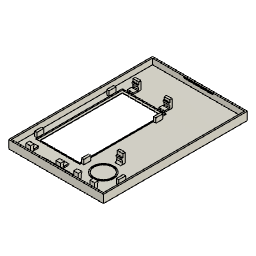
epaper Outer Case Top (Autodesk Fusion 360 design; units mm, degrees)
Autodesk Fusion 360 part; units mm, degrees
sketch "Sketch2" plane through (0, 0, 0) normal (0, 0, 1) x (1, 0, 0)
  line L0 (0, 0) -> (82, 0)
  line L1 (82, 0) -> (82, 124.4)
  line L2 (82, 124.4) -> (0, 124.4)
  line L3 (0, 124.4) -> (0, 0)
  dimension "d135" = 124.4
  dimension "d136" = 82
  constraint horizontal L0
  constraint vertical L1
  constraint horizontal L2
  constraint vertical L3
  constraint coincident L0.start L3.end
  measures "d135" distance of L0.start L2.end
  measures "d136" distance of L0.start L0.end
extrude "Extrude4" add sketch "Sketch2" along normal blind 2
sketch "Sketch3" plane through (0, 0, 2) normal (0, 0, 1) x (-1, 0, 0)
  line L0 (0, -124.4) -> (0, 0)
  line L1 (0, 0) -> (-82, 0)
  line L2 (-82, 0) -> (-82, -124.4)
  line L3 (-82, -124.4) -> (0, -124.4)
  line L4 (-1.25, -1.25) -> (-80.75, -1.25)
  line L5 (-80.75, -1.25) -> (-80.75, -123.15)
  line L6 (-80.75, -123.15) -> (-1.25, -123.15)
  line L7 (-1.25, -123.15) -> (-1.25, -1.25)
  line L8 (-51.575, -4.675) -> (-55.575, -4.675)
  line L9 (-55.575, -4.675) -> (-55.575, -7.175)
  line L10 (-55.575, -7.175) -> (-51.575, -7.175)
  line L11 (-51.575, -7.175) -> (-51.575, -4.675)
  line L12 (-65.625, -4.675) -> (-69.625, -4.675)
  line L13 (-69.625, -4.675) -> (-69.625, -7.175)
  line L14 (-69.625, -7.175) -> (-65.625, -7.175)
  line L15 (-65.625, -7.175) -> (-65.625, -4.675)
  line L16 (-58.1, -35.275) -> (-63.1, -35.275)
  line L17 (-63.1, -35.275) -> (-63.1, -37.775)
  line L18 (-63.1, -37.775) -> (-58.1, -37.775)
  line L19 (-58.1, -37.775) -> (-58.1, -35.275)
  line L20 (-74.75, -24.5) -> (-76.75, -24.5)
  line L21 (-76.75, -24.5) -> (-76.75, -18.5)
  line L22 (-76.75, -18.5) -> (-74.75, -18.5)
  line L23 (-74.75, -18.5) -> (-74.75, -24.5)
  line L24 (-44.45, -24.5) -> (-46.45, -24.5)
  line L25 (-46.45, -24.5) -> (-46.45, -18.5)
  line L26 (-46.45, -18.5) -> (-44.45, -18.5)
  line L27 (-44.45, -18.5) -> (-44.45, -24.5)
  circle A0 centre (-60.6, -21.25) radius 8.0623
  circle A1 centre (-60.6, -21.25) radius 9.0623
  line L28 (0, 0) -> (-82, 0)
  line L29 (0, -124.4) -> (0, 0)
  line L30 (-80.75, -110) -> (-80.75, -72)
  line L31 (-46.45, -80.825) -> (-44.45, -80.825)
  line L32 (-44.45, -80.825) -> (-44.45, -86.825)
  line L33 (-44.45, -86.825) -> (-46.45, -86.825)
  line L34 (-46.45, -86.825) -> (-46.45, -80.825)
  line L35 (-3.95, -86.825) -> (-5.95, -86.825)
  line L36 (-5.95, -86.825) -> (-5.95, -80.825)
  line L37 (-5.95, -80.825) -> (-3.95, -80.825)
  line L38 (-3.95, -80.825) -> (-3.95, -86.825)
  line L39 (-3.95, -24.5) -> (-5.95, -24.5)
  line L40 (-5.95, -24.5) -> (-5.95, -18.5)
  line L41 (-5.95, -18.5) -> (-3.95, -18.5)
  line L42 (-3.95, -18.5) -> (-3.95, -24.5)
  line L43 (-10.2, -7.175) -> (-14.2, -7.175)
  line L44 (-14.2, -7.175) -> (-14.2, -4.675)
  line L45 (-14.2, -4.675) -> (-10.2, -4.675)
  line L46 (-10.2, -4.675) -> (-10.2, -7.175)
  line L47 (-36.2, -7.175) -> (-40.2, -7.175)
  line L48 (-40.2, -7.175) -> (-40.2, -4.675)
  line L49 (-40.2, -4.675) -> (-36.2, -4.675)
  line L50 (-36.2, -4.675) -> (-36.2, -7.175)
  line L51 (-10.2, -99.325) -> (-15.2, -99.325)
  line L52 (-15.2, -99.325) -> (-15.2, -97.075)
  line L53 (-15.2, -97.075) -> (-10.2, -97.075)
  line L54 (-10.2, -97.075) -> (-10.2, -99.325)
  line L55 (-37.2, -99.325) -> (-42.2, -99.325)
  line L56 (-42.2, -99.325) -> (-42.2, -97.075)
  line L57 (-42.2, -97.075) -> (-37.2, -97.075)
  line L58 (-37.2, -97.075) -> (-37.2, -99.325)
  line L59 (-10.2, -8.175) -> (-14.2, -8.175)
  line L60 (-14.2, -8.175) -> (-14.2, -11.675)
  line L61 (-14.2, -11.675) -> (-10.2, -11.675)
  line L62 (-10.2, -11.675) -> (-10.2, -8.175)
  line L63 (-40.2, -8.175) -> (-36.2, -8.175)
  line L64 (-36.2, -8.175) -> (-36.2, -11.675)
  line L65 (-36.2, -11.675) -> (-40.2, -11.675)
  line L66 (-40.2, -11.675) -> (-40.2, -8.175)
  line L67 (-10.2, -96.075) -> (-15.2, -96.075)
  line L68 (-15.2, -96.075) -> (-15.2, -92.575)
  line L69 (-15.2, -92.575) -> (-10.2, -92.575)
  line L70 (-10.2, -92.575) -> (-10.2, -96.075)
  line L71 (-42.2, -96.075) -> (-37.2, -96.075)
  line L72 (-37.2, -96.075) -> (-37.2, -92.575)
  line L73 (-37.2, -92.575) -> (-42.2, -92.575)
  line L74 (-42.2, -92.575) -> (-42.2, -96.075)
  line L75 (-8.2, -90.175) -> (-42.2, -90.175)
  line L76 (-42.2, -90.175) -> (-42.2, -19.175)
  line L77 (-42.2, -19.175) -> (-8.2, -19.175)
  line L78 (-8.2, -19.175) -> (-8.2, -90.175)
  line L79 (-6.2, -17.175) -> (-6.2, -92.175)
  line L80 (-6.2, -92.175) -> (-44.2, -92.175)
  line L81 (-44.2, -92.175) -> (-44.2, -17.175)
  line L82 (-44.2, -17.175) -> (-6.2, -17.175)
  dimension "d82" = -1.25
  dimension "d87" = 4
  dimension "d88" = 2.5
  dimension "d89" = 4
  dimension "d90" = 2.5
  dimension "d93" = 5
  dimension "d94" = 2.5
  dimension "d96" = 2
  dimension "d97" = 6
  dimension "d98" = 2
  dimension "d99" = 6
  dimension "d102" = 11.65
  dimension "d103" = 28.3
  dimension "d104" = 1
  dimension "d122" = 14.15
  dimension "d129" = 79.5
  dimension "d131" = 20
  dimension "d137" = 82
  dimension "d169" = 28.1
  dimension "d170" = 14.025
  dimension "d193" = 124.4
  dimension "d213" = 20.15
  dimension "d216" = 5.025
  dimension "d217" = 10.05
  dimension "d222" = 2
  dimension "d223" = 6
  dimension "d224" = 2
  dimension "d225" = 6
  dimension "d226" = 2
  dimension "d227" = 6
  dimension "d228" = 38.5
  dimension "d229" = 22
  dimension "d230" = 8.25
  dimension "d231" = 2.5
  dimension "d232" = 2.5
  dimension "d234" = 5
  dimension "d235" = 2.25
  dimension "d236" = 89.9
  dimension "d237" = 4
  dimension "d238" = 4
  dimension "d239" = 2.25
  dimension "d240" = 5
  dimension "d241" = 22
  dimension "d242" = 10.25
  dimension "d243" = 4
  dimension "d244" = 3.5
  dimension "d245" = 4
  dimension "d246" = 3.5
  dimension "d247" = 5
  dimension "d248" = 3.5
  dimension "d249" = 5
  dimension "d250" = 3.5
  dimension "d251" = 1
  dimension "d252" = 1
  dimension "d257" = 34
  dimension "d258" = 71
  dimension "d259" = 12
  dimension "d260" = 2.25
  dimension "d263" = -2
  constraint horizontal L8
  constraint vertical L9
  constraint horizontal L10
  constraint vertical L11
  constraint horizontal L12
  constraint vertical L13
  constraint horizontal L14
  constraint vertical L15
  constraint horizontal L16
  constraint vertical L17
  constraint horizontal L18
  constraint vertical L19
  constraint horizontal L10.end L14.end
  constraint horizontal L20
  constraint vertical L21
  constraint horizontal L22
  constraint vertical L23
  constraint horizontal L24
  constraint vertical L25
  constraint horizontal L26
  constraint vertical L27
  constraint horizontal L20.start L24.end
  constraint vertical L30
  constraint coincident L5 L30.end
  constraint horizontal L31
  constraint vertical L32
  constraint horizontal L33
  constraint vertical L34
  constraint collinear L27 L32
  constraint horizontal L35
  constraint vertical L36
  constraint horizontal L37
  constraint vertical L38
  constraint horizontal L39
  constraint vertical L40
  constraint horizontal L41
  constraint vertical L42
  constraint collinear L38 L42
  constraint collinear L24 L39
  constraint collinear L33 L35
  constraint horizontal L43
  constraint vertical L44
  constraint horizontal L45
  constraint vertical L46
  constraint horizontal L47
  constraint vertical L48
  constraint horizontal L49
  constraint vertical L50
  constraint collinear L43 L47
  constraint horizontal L51
  constraint vertical L52
  constraint horizontal L53
  constraint vertical L54
  constraint collinear L46 L54
  constraint horizontal L55
  constraint vertical L56
  constraint horizontal L57
  constraint vertical L58
  constraint collinear L51 L55
  constraint horizontal L59
  constraint vertical L60
  constraint horizontal L61
  constraint vertical L62
  constraint horizontal L63
  constraint vertical L64
  constraint horizontal L65
  constraint vertical L66
  constraint horizontal L67
  constraint vertical L68
  constraint horizontal L69
  constraint vertical L70
  constraint horizontal L71
  constraint vertical L72
  constraint horizontal L73
  constraint vertical L74
  constraint collinear L67 L71
  constraint collinear L59 L63
  constraint collinear L46 L62
  constraint collinear L48 L66
  constraint collinear L54 L70
  constraint collinear L56 L74
  constraint horizontal L75
  constraint vertical L76
  constraint horizontal L77
  constraint vertical L78
  constraint collinear L8 L45
  measures "d87" distance of L8.start L8.end
  measures "d88" distance of L8.start L10.end
  measures "d89" distance of L12.start L12.end
  measures "d90" distance of L12.start L14.end
  measures "d93" distance of L16.start L16.end
  measures "d94" distance of L16.start L18.end
  measures "d96" distance of L20.start L20.end
  measures "d97" distance of L20.start L22.end
  measures "d98" distance of L24.start L24.end
  measures "d99" distance of L24.start L26.end
  measures "d102" distance of L17 L23
  measures "d103" distance of L23 L25
  measures "d122" distance of L25 A0.centre
  measures "d129" distance of L5 L7
  measures "d131" distance of L4 A0.centre
  measures "d137" distance of L0.end L1.end
  measures "d169" distance of L14 L16
  measures "d170" distance of L16 A0.centre
  measures "d193" distance of L0.start L0.end
  measures "d213" distance of L5 A0.centre
  measures "d216" distance of L9 A0.centre
  measures "d217" distance of L9 L15
  measures "d222" distance of L31.start L31.end
  measures "d223" distance of L31.start L33.end
  measures "d224" distance of L35.start L35.end
  measures "d225" distance of L35.start L37.end
  measures "d226" distance of L39.start L39.end
  measures "d227" distance of L39.start L41.end
  measures "d228" distance of L32 L36
  measures "d229" distance of L44 L50
  measures "d230" distance of L27 L50
  measures "d231" distance of L43.start L45.end
  measures "d232" distance of L47.end L48.end
  measures "d234" distance of L51.start L51.end
  measures "d235" distance of L51.start L53.end
  measures "d236" distance of L43 L53
  measures "d237" distance of L44.end L45.end
  measures "d238" distance of L48.end L49.end
  measures "d239" distance of L55.start L57.end
  measures "d240" distance of L55.start L55.end
  measures "d241" distance of L52 L58
  measures "d242" distance of L33 L56.end
  measures "d243" distance of L59.start L59.end
  measures "d244" distance of L59.start L61.end
  measures "d245" distance of L63.start L63.end
  measures "d246" distance of L63.start L65.end
  measures "d247" distance of L67.start L67.end
  measures "d248" distance of L67.start L69.end
  measures "d249" distance of L71.start L71.end
  measures "d250" distance of L71.start L73.end
  measures "d251" distance of L53 L67
  measures "d252" distance of L43 L59
  measures "d257" distance of L76 L78
  measures "d258" distance of L75 L77
  measures "d259" distance of L43 L77
  measures "d260" distance of L36 L78
extrude "Extrude26" cut sketch "Sketch3" against normal blind 1 contours L79 L80 L81 L82
extrude "Extrude25" cut sketch "Sketch3" against normal blind 4 contours L75 L76 L77 L78
extrude "Extrude24" add sketch "Sketch3" along normal blind 3 contours L43 L44 L45 L46 | L47 L48 L49 L50 | L51 L52 L53 L54 | L55 L56 L57 L58
extrude "Extrude23" add sketch "Sketch3" along normal blind 1.2 contours L59 L60 L61 L62 | L63 L64 L65 L66 | L67 L68 L69 L70 | L71 L72 L73 L74
extrude "Extrude11" add sketch "Sketch3" along normal blind 0.3 contours A1
extrude "Extrude12" add sketch "Sketch3" along normal blind 4 contours L20 L21 L22 L23 | L24 L25 L26 L27 | L31 L32 L33 L34 | L35 L36 L37 L38 | L39 L40 L41 L42
extrude "Extrude13" add sketch "Sketch3" along normal blind 3.23 contours L8 L9 L10 L11 | L12 L13 L14 L15 | L16 L17 L18 L19
sketch "Sketch7" plane through (0, 0, 5.23) normal (0, 0, 1) x (-1, 0, 0)
  line L0 (-58.1, -37.775) -> (-63.1, -37.775)
  line L1 (-63.1, -37.775) -> (-63.1, -34.775)
  line L2 (-63.1, -34.775) -> (-58.1, -34.775)
  line L3 (-58.1, -34.775) -> (-58.1, -37.775)
  line L4 (-51.575, -4.675) -> (-55.575, -4.675)
  line L5 (-55.575, -4.675) -> (-55.575, -7.675)
  line L6 (-55.575, -7.675) -> (-51.575, -7.675)
  line L7 (-51.575, -7.675) -> (-51.575, -4.675)
  line L8 (-65.625, -4.675) -> (-69.625, -4.675)
  line L9 (-69.625, -4.675) -> (-69.625, -7.675)
  line L10 (-69.625, -7.675) -> (-65.625, -7.675)
  line L11 (-65.625, -7.675) -> (-65.625, -4.675)
  line L12 (-58.1, -37.775) -> (-58.1, -35.275)
  line L13 (-58.1, -35.275) -> (-63.1, -35.275)
  line L14 (-63.1, -35.275) -> (-63.1, -37.775)
  line L15 (-63.1, -37.775) -> (-58.1, -37.775)
  line L16 (-65.625, -7.175) -> (-65.625, -4.675)
  line L17 (-65.625, -4.675) -> (-69.625, -4.675)
  line L18 (-69.625, -4.675) -> (-69.625, -7.175)
  line L19 (-69.625, -7.175) -> (-65.625, -7.175)
  line L20 (-51.575, -7.175) -> (-51.575, -4.675)
  line L21 (-51.575, -4.675) -> (-55.575, -4.675)
  line L22 (-55.575, -4.675) -> (-55.575, -7.175)
  line L23 (-55.575, -7.175) -> (-51.575, -7.175)
  point P0 (-58.1, -37.775)
  point P1 (-51.575, -4.675)
  point P2 (-65.625, -4.675)
  point P3 (-63.1, -37.775)
  dimension "d112" = 3
  dimension "d113" = 4
  dimension "d114" = 3
  dimension "d115" = 4
  dimension "d116" = 3
  constraint horizontal L0
  constraint vertical L1
  constraint horizontal L2
  constraint vertical L3
  constraint horizontal L4
  constraint vertical L5
  constraint horizontal L6
  constraint vertical L7
  constraint horizontal L8
  constraint vertical L9
  constraint horizontal L10
  constraint vertical L11
  constraint coincident P0 L0.start
  constraint coincident P1 L4.start
  constraint coincident P2 L8.start
  constraint coincident P3 L0.end
  measures "d112" distance of P0 L2.end
  measures "d113" distance of P1 L4.end
  measures "d114" distance of P1 L6.end
  measures "d115" distance of P2 L8.end
  measures "d116" distance of P2 L10.end
extrude "Extrude14" add sketch "Sketch7" along normal blind 1.8
extrude "Extrude10" add sketch "Sketch3" along normal blind 5 contours L0 L1 L2 L3 L28 L29
sketch "Sketch12" plane through (0, 0, 7.03) normal (0, 0, 1) x (-1, 0, 0)
  line L0 (-58.1, -34.775) -> (-63.1, -34.775)
  line L1 (-63.1, -34.775) -> (-63.1, -37.775)
  line L2 (-63.1, -37.775) -> (-58.1, -37.775)
  line L3 (-58.1, -37.775) -> (-58.1, -34.775)
  line L4 (-58.1, -37.775) -> (-63.1, -37.775)
  line L5 (-63.1, -37.775) -> (-63.1, -35.775)
  line L6 (-63.1, -35.775) -> (-58.1, -35.775)
  line L7 (-58.1, -35.775) -> (-58.1, -37.775)
  dimension "d160" = 2
  constraint horizontal L4
  constraint vertical L5
  constraint horizontal L6
  constraint vertical L7
  constraint coincident L2.end L3.start
  constraint coincident L1.end L2.start
  measures "d160" distance of L2.end L6.end
extrude "Extrude18" add sketch "Sketch12" along normal blind 3 contours L1 L2 L3 L4 L5 L6 L7
chamfer "Chamfer5" distance 0.5 angle 45 3 edges at (60.6, 34.775, 5.23) (53.575, 7.675, 5.23) (67.625, 7.675, 5.23)
sketch "Sketch19" plane through (0, 0, 5) normal (0, 0, 1) x (-1, 0, 0)
  line L0 (-10.2, -4.675) -> (-14.2, -4.675)
  line L1 (-14.2, -4.675) -> (-14.2, -7.175)
  line L2 (-14.2, -7.175) -> (-10.2, -7.175)
  line L3 (-10.2, -7.175) -> (-10.2, -4.675)
  line L4 (-10.2, -4.675) -> (-14.2, -4.675)
  line L5 (-14.2, -4.675) -> (-14.2, -7.775)
  line L6 (-14.2, -7.775) -> (-10.2, -7.775)
  line L7 (-10.2, -7.775) -> (-10.2, -4.675)
  dimension "d267" = 4
  dimension "d268" = 3.1
  constraint horizontal L4
  constraint vertical L5
  constraint horizontal L6
  constraint vertical L7
  constraint coincident L0.start L3.end
  measures "d267" distance of L0.start L0.end
  measures "d268" distance of L0.start L6.end
extrude "Extrude27" add sketch "Sketch19" along normal blind 2
sketch "Sketch20" plane through (0, 0, 5) normal (0, 0, 1) x (-1, 0, 0)
  line L0 (-36.2, -4.675) -> (-40.2, -4.675)
  line L1 (-40.2, -4.675) -> (-40.2, -7.175)
  line L2 (-40.2, -7.175) -> (-36.2, -7.175)
  line L3 (-36.2, -7.175) -> (-36.2, -4.675)
  line L4 (-36.2, -4.675) -> (-40.2, -4.675)
  line L5 (-40.2, -4.675) -> (-40.2, -7.775)
  line L6 (-40.2, -7.775) -> (-36.2, -7.775)
  line L7 (-36.2, -7.775) -> (-36.2, -4.675)
  dimension "d271" = 4
  dimension "d272" = 3.1
  constraint horizontal L4
  constraint vertical L5
  constraint horizontal L6
  constraint vertical L7
  constraint coincident L0.start L3.end
  measures "d271" distance of L0.start L0.end
  measures "d272" distance of L0.start L6.end
extrude "Extrude28" add sketch "Sketch20" along normal blind 2
sketch "Sketch21" plane through (0, 0, 5) normal (0, 0, 1) x (-1, 0, 0)
  line L0 (-10.2, -97.075) -> (-15.2, -97.075)
  line L1 (-15.2, -97.075) -> (-15.2, -99.325)
  line L2 (-15.2, -99.325) -> (-10.2, -99.325)
  line L3 (-10.2, -99.325) -> (-10.2, -97.075)
  line L4 (-10.2, -99.325) -> (-15.2, -99.325)
  line L5 (-15.2, -99.325) -> (-15.2, -96.475)
  line L6 (-15.2, -96.475) -> (-10.2, -96.475)
  line L7 (-10.2, -96.475) -> (-10.2, -99.325)
  dimension "d275" = 5
  dimension "d276" = 2.85
  constraint horizontal L4
  constraint vertical L5
  constraint horizontal L6
  constraint vertical L7
  constraint coincident L2.end L3.start
  measures "d275" distance of L2.end L1.end
  measures "d276" distance of L2.end L6.end
extrude "Extrude29" add sketch "Sketch21" along normal blind 2
sketch "Sketch22" plane through (0, 0, 5) normal (0, 0, 1) x (-1, 0, 0)
  line L0 (-37.2, -97.075) -> (-42.2, -97.075)
  line L1 (-42.2, -97.075) -> (-42.2, -99.325)
  line L2 (-42.2, -99.325) -> (-37.2, -99.325)
  line L3 (-37.2, -99.325) -> (-37.2, -97.075)
  line L4 (-37.2, -99.325) -> (-42.2, -99.325)
  line L5 (-42.2, -99.325) -> (-42.2, -96.475)
  line L6 (-42.2, -96.475) -> (-37.2, -96.475)
  line L7 (-37.2, -96.475) -> (-37.2, -99.325)
  dimension "d279" = 5
  dimension "d280" = 2.85
  constraint horizontal L4
  constraint vertical L5
  constraint horizontal L6
  constraint vertical L7
  constraint coincident L2.end L3.start
  measures "d279" distance of L2.end L1.end
  measures "d280" distance of L2.end L6.end
extrude "Extrude30" add sketch "Sketch22" along normal blind 2
chamfer "Chamfer9" distance 0.6 angle 45 2 edges at (12.2, 7.775, 5) (38.2, 7.775, 5)
chamfer "Chamfer10" distance 0.6 angle 45 2 edges at (12.7, 96.475, 5) (39.7, 96.475, 5)
sketch "Sketch23" plane through (0, 0, 7) normal (0, 0, 1) x (-1, 0, 0)
  line L0 (-10.2, -96.475) -> (-15.2, -96.475)
  line L1 (-15.2, -96.475) -> (-15.2, -99.325)
  line L2 (-15.2, -99.325) -> (-10.2, -99.325)
  line L3 (-10.2, -99.325) -> (-10.2, -96.475)
  line L4 (-10.2, -99.325) -> (-15.2, -99.325)
  line L5 (-15.2, -99.325) -> (-15.2, -97.325)
  line L6 (-15.2, -97.325) -> (-10.2, -97.325)
  line L7 (-10.2, -97.325) -> (-10.2, -99.325)
  dimension "d284" = 5
  dimension "d285" = 2
  constraint horizontal L4
  constraint vertical L5
  constraint horizontal L6
  constraint vertical L7
  constraint coincident L2.end L3.start
  measures "d284" distance of L2.end L1.end
  measures "d285" distance of L2.end L6.end
extrude "Extrude31" add sketch "Sketch23" along normal blind 2 contours L1 L2 L3 L4 L5 L6 L7
sketch "Sketch24" plane through (0, 0, 7) normal (0, 0, 1) x (-1, 0, 0)
  line L0 (-37.2, -96.475) -> (-42.2, -96.475)
  line L1 (-42.2, -96.475) -> (-42.2, -99.325)
  line L2 (-42.2, -99.325) -> (-37.2, -99.325)
  line L3 (-37.2, -99.325) -> (-37.2, -96.475)
  line L4 (-37.2, -99.325) -> (-42.2, -99.325)
  line L5 (-42.2, -99.325) -> (-42.2, -97.325)
  line L6 (-42.2, -97.325) -> (-37.2, -97.325)
  line L7 (-37.2, -97.325) -> (-37.2, -99.325)
  dimension "d288" = 5
  dimension "d289" = 2
  constraint horizontal L4
  constraint vertical L5
  constraint horizontal L6
  constraint vertical L7
  constraint coincident L2.end L3.start
  measures "d288" distance of L2.end L1.end
  measures "d289" distance of L2.end L6.end
extrude "Extrude32" add sketch "Sketch24" along normal blind 2 contours L1 L2 L3 L4 L5 L6 L7
sketch "Sketch8" plane through (0, 0, 0) normal (0, 0, -1) x (1, 0, 0)
  line L0 (0, 0) -> (0, -124.4)
  line L1 (0, -124.4) -> (82, -124.4)
  line L2 (82, -124.4) -> (82, 0)
  line L3 (82, 0) -> (0, 0)
  line L4 (57.8279, -10.7958) -> (57.8279, -104.0301) construction
  line L5 (57.8279, -104.0301) -> (69.8279, -104.0301) construction
  line L6 (69.8279, -104.0301) -> (69.8279, -10.7958) construction
  line L7 (69.8279, -10.7958) -> (57.8279, -10.7958) construction
  line L8 (42.2, -19.175) -> (42.2, -90.175)
  line L9 (42.2, -90.175) -> (8.2, -90.175)
  line L10 (8.2, -90.175) -> (8.2, -19.175)
  line L11 (8.2, -19.175) -> (42.2, -19.175)
  text T0 "Ferg Data Logger" font "Arial" height 12 align ink ink in box 0 x 0 at (57.8279, -10.7958) x (0, -1) y (1, 0) spacing 1 height is em
  constraint perpendicular L4 L5
  constraint parallel L4 L6
  constraint parallel L5 L7
extrude "Extrude16" cut sketch "Sketch8" against normal blind 0.5 text T0
sketch "Sketch10" plane through (0, 123.15, 0) normal (0, -1, 0) x (1, 0, 0)
  line L0 (1.25, 2) -> (80.75, 2)
  line L1 (80.75, 2) -> (80.75, 7)
  line L2 (80.75, 7) -> (1.25, 7)
  line L3 (1.25, 7) -> (1.25, 2)
  line L4 (28.5, 7) -> (53.5, 7)
  line L5 (53.5, 7) -> (53.5, 5.6)
  line L6 (53.5, 5.6) -> (28.5, 5.6)
  line L7 (28.5, 5.6) -> (28.5, 7)
  dimension "d139" = 25
  dimension "d140" = 1.4
  dimension "d141" = 79.5
  dimension "d142" = 27.25
  constraint horizontal L4
  constraint vertical L5
  constraint horizontal L6
  constraint vertical L7
  constraint coincident L2 L4.start
  measures "d139" distance of L4.start L4.end
  measures "d140" distance of L4.start L6.end
  measures "d141" distance of L1.end L2.end
  measures "d142" distance of L3 L7
revolve "Revolve1" add sketch "Sketch10" angle 25 about axis through (53.5, 123.15, 5.6) along (1, 0, 0) contours L2 L4 L5 L6 L7
sketch "Sketch11" plane through (0, 1.25, 0) normal (0, 1, 0) x (-1, 0, 0)
  line L0 (-80.75, 2) -> (-1.25, 2)
  line L1 (-1.25, 2) -> (-1.25, 7)
  line L2 (-1.25, 7) -> (-80.75, 7)
  line L3 (-53.5, 7) -> (-28.5, 7)
  line L4 (-28.5, 7) -> (-28.5, 5.6)
  line L5 (-28.5, 5.6) -> (-53.5, 5.6)
  line L6 (-53.5, 5.6) -> (-53.5, 7)
  line L7 (-80.75, 7) -> (-80.75, 2)
  dimension "d144" = 25
  dimension "d145" = 1.4
  dimension "d146" = 79.5
  dimension "d147" = 27.25
  constraint horizontal L3
  constraint vertical L4
  constraint horizontal L5
  constraint vertical L6
  constraint coincident L2 L3.start
  measures "d144" distance of L3.start L3.end
  measures "d145" distance of L3.start L5.end
  measures "d146" distance of L1.end L2.end
  measures "d147" distance of L1 L4
revolve "Revolve2" add sketch "Sketch11" angle 25 about axis through (28.5, 1.25, 5.6) along (-1, 0, 0) contours L2 L3 L4 L5 L6
fillet "Fillet3" radius 1.5 1 edges at (60.6, 35.275, 2)
fillet "Fillet3" radius 1.5 2 edges at (12.7, 97.075, 2) (39.7, 97.075, 2)
fillet "Fillet3" radius 1.5 2 edges at (12.2, 7.175, 2) (38.2, 7.175, 2)
sketch "Sketch18" plane through (0, 0, 2) normal (0, 0, 1) x (-1, 0, 0)
  line L0 (-58.1, -33.775) -> (-58.1, -37.775)
  line L1 (-58.1, -37.775) -> (-63.1, -37.775)
  line L2 (-63.1, -37.775) -> (-63.1, -33.775)
  line L3 (-63.1, -33.775) -> (-58.1, -33.775)
  line L4 (-1.25, -1.25) -> (-80.75, -1.25)
  line L5 (-80.75, -1.25) -> (-80.75, -123.15)
  line L6 (-80.75, -123.15) -> (-1.25, -123.15)
  line L7 (-1.25, -123.15) -> (-1.25, -1.25)
  line L8 (-65.625, -7.175) -> (-69.625, -7.175)
  line L9 (-69.625, -7.175) -> (-69.625, -4.675)
  line L10 (-69.625, -4.675) -> (-65.625, -4.675)
  line L11 (-65.625, -4.675) -> (-65.625, -7.175)
  line L12 (-51.575, -7.175) -> (-55.575, -7.175)
  line L13 (-55.575, -7.175) -> (-55.575, -4.675)
  line L14 (-55.575, -4.675) -> (-51.575, -4.675)
  line L15 (-51.575, -4.675) -> (-51.575, -7.175)
  line L16 (-74.75, -18.5) -> (-74.75, -24.5)
  line L17 (-74.75, -24.5) -> (-76.75, -24.5)
  line L18 (-76.75, -24.5) -> (-76.75, -18.5)
  line L19 (-76.75, -18.5) -> (-74.75, -18.5)
  line L20 (-44.45, -18.5) -> (-44.45, -24.5)
  line L21 (-44.45, -24.5) -> (-46.45, -24.5)
  line L22 (-46.45, -24.5) -> (-46.45, -18.5)
  line L23 (-46.45, -18.5) -> (-44.45, -18.5)
  circle A0 centre (-60.6, -21.25) radius 9.0623
  line L24 (-5.2392, -108.6182) -> (-65.3716, -108.6182)
  line L25 (-65.3716, -108.6182) -> (-65.3716, -3.4636)
  line L26 (-65.3716, -3.4636) -> (-5.2392, -3.4636)
  line L27 (-5.2392, -3.4636) -> (-5.2392, -108.6182)
  line L28 (-46.45, -86.825) -> (-46.45, -80.825)
  line L29 (-46.45, -80.825) -> (-44.45, -80.825)
  line L30 (-44.45, -80.825) -> (-44.45, -86.825)
  line L31 (-44.45, -86.825) -> (-46.45, -86.825)
  line L32 (-3.95, -80.825) -> (-3.95, -86.825)
  line L33 (-3.95, -86.825) -> (-5.95, -86.825)
  line L34 (-5.95, -86.825) -> (-5.95, -80.825)
  line L35 (-5.95, -80.825) -> (-3.95, -80.825)
  line L36 (-3.95, -18.5) -> (-3.95, -24.5)
  line L37 (-3.95, -24.5) -> (-5.95, -24.5)
  line L38 (-5.95, -24.5) -> (-5.95, -18.5)
  line L39 (-5.95, -18.5) -> (-3.95, -18.5)
  line L40 (-42.2, -92.575) -> (-37.2, -92.575)
  line L41 (-37.2, -92.575) -> (-37.2, -96.075)
  line L42 (-42.2, -96.075) -> (-42.2, -92.575)
  line L43 (-10.2, -11.675) -> (-14.2, -11.675)
  line L44 (-14.2, -11.675) -> (-14.2, -8.175)
  line L45 (-10.2, -8.175) -> (-10.2, -11.675)
  line L46 (-10.2, -92.575) -> (-10.2, -96.075)
  line L47 (-15.2, -96.075) -> (-15.2, -92.575)
  line L48 (-15.2, -92.575) -> (-10.2, -92.575)
  line L49 (-40.2, -11.675) -> (-40.2, -8.175)
  line L50 (-36.2, -8.175) -> (-36.2, -11.675)
  line L51 (-36.2, -11.675) -> (-40.2, -11.675)
  line L52 (-37.2, -96.075) -> (-37.2, -99.325)
  line L53 (-37.2, -99.325) -> (-42.2, -99.325)
  line L54 (-42.2, -99.325) -> (-42.2, -96.075)
  line L55 (-10.2, -4.675) -> (-10.2, -8.175)
  line L56 (-14.2, -8.175) -> (-14.2, -4.675)
  line L57 (-14.2, -4.675) -> (-10.2, -4.675)
  line L58 (-10.2, -96.075) -> (-10.2, -99.325)
  line L59 (-10.2, -99.325) -> (-15.2, -99.325)
  line L60 (-15.2, -99.325) -> (-15.2, -96.075)
  line L61 (-36.2, -4.675) -> (-36.2, -8.175)
  line L62 (-40.2, -8.175) -> (-40.2, -4.675)
  line L63 (-40.2, -4.675) -> (-36.2, -4.675)
  line L64 (-6.2, -92.175) -> (-44.2, -92.175)
  line L65 (-44.2, -92.175) -> (-44.2, -17.175)
  line L66 (-44.2, -17.175) -> (-6.2, -17.175)
  line L67 (-6.2, -17.175) -> (-6.2, -92.175)
  constraint horizontal L24
  constraint vertical L25
  constraint horizontal L26
  constraint vertical L27
extrude "Extrude22" [suppressed]
chamfer "Chamfer8" distance 0.75 angle 45 4 edges at (25.2, 19.175, 0) (8.2, 54.675, 0) (42.2, 54.675, 0) (25.2, 90.175, 0)
equation "d87 = d89"
equation "d88 = d94"
equation "d90 = d94"
equation "d96 = d98"
equation "d97 = d99"
equation "d102 = ( d103 - d93 ) / 2"
equation "d109 = 2.93 mm + 0.3 mm"
equation "d112 = d114"
equation "d115 = d113"
equation "d116 = d114"
equation "d122 = d103 / 2"
equation "d142 = ( 79.50 mm - d139 ) / 2"
equation "d147 = ( 79.50 mm - d144 ) / 2"
equation "d213 = 17.15 mm + 1.5 mm + 1.5 mm"
equation "d222 = d98"
equation "d223 = d99"
equation "d224 = d98"
equation "d225 = d99"
equation "d226 = d98"
equation "d227 = d99"
equation "d230 = ( d228 - d229 ) / 2"
equation "d232 = d231"
equation "d234 = d93"
equation "d237 = d238"
equation "d238 = d89"
equation "d239 = d235"
equation "d240 = d234"
equation "d241 = d229"
equation "d244 = d248"
equation "d246 = d244"
equation "d247 = d234"
equation "d249 = d240"
equation "d250 = d248"
equation "d255 = 1.3 mm + 1.7 mm"
equation "d260 = ( d228 - d257 ) / 2"
